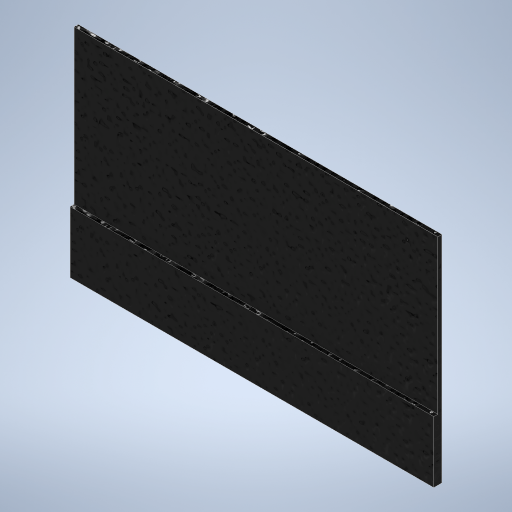
# Autodesk Inventor part: монитор
Saved by Autodesk Inventor 2023 (Build 270158000, 158)
## iProperties
Created: 2025-02-04
Part Number: монитор
Material: Типовые
Document SubType Name: Modeling
Designer: baranovaem
Density: 1 g/cm^3
Appearance: Черный
Author: baranovaem
Autodesk Inventor part; units mm, degrees
ref_plane "YZ Plane" through (0, 0, 0) normal (1, 0, 0) x (0, 1, 0)
ref_plane "XZ Plane" through (0, 0, 0) normal (0, 1, 0) x (-1, 0, 0)
ref_plane "XY Plane" through (0, 0, 0) normal (0, 0, 1) x (1, 0, 0)
sketch "Эскиз1" plane through (0, 0, 0) normal (0, 0, 1) x (1, 0, 0)
  line L0 (-177.5, 105) -> (177.5, 105)
  line L1 (177.5, 105) -> (177.5, -105)
  line L2 (177.5, -105) -> (-177.5, -105)
  line L3 (-177.5, -105) -> (-177.5, 105)
  line L4 (-177.5, 105) -> (177.5, -105) construction
  line L5 (177.5, 105) -> (-177.5, -105) construction
  point P0 (0, 0)
  dimension "d0" = 355
  dimension "d1" = 210
  constraints: 12 end point, 2 midpoint, 2 parallel, 1 horizontal, 1 perpendicular
  measures "d0" distance of L1.end L2.end
  measures "d1" distance of L0.end L1.end
extrude "Выдавливание1" add sketch "Эскиз1" along normal blind 4
sketch "Эскиз2" plane through (0, 0, 4) normal (0, 0, 1) x (1, 0, 0)
  line L0 (-177.5, -105) -> (177.5, -105) projected
  line L1 (177.5, -105) -> (177.5, 105) projected
  line L2 (-177.5, -105) -> (177.5, -105)
  line L3 (177.5, -105) -> (177.5, -45)
  line L4 (177.5, -45) -> (-177.5, -45)
  line L5 (-177.5, -45) -> (-177.5, -105)
  point P0 (0, 0)
  dimension "d4" = 60
  constraints: 8 end point, 2 parallel, 1 horizontal, 1 perpendicular, 1 point on line
  measures "d4" distance between parallel lines of L0 L4
extrude "Выдавливание2" add sketch "Эскиз2" along normal blind 4
